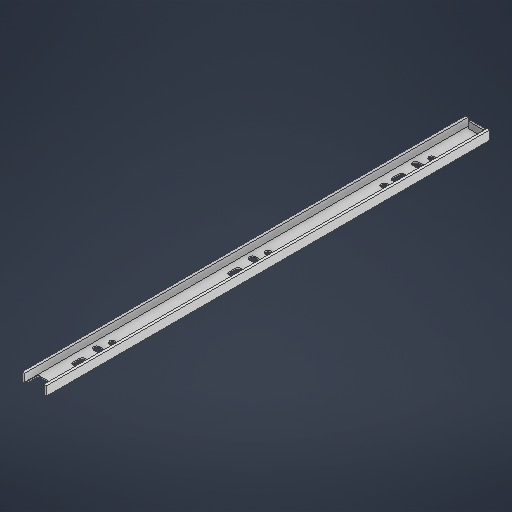
# Autodesk Inventor part: 3 часть направляшки 35
Saved by Autodesk Inventor 2025 (Build 290162000, 162)
## iProperties
Created: 2024-11-23
Part Number: 3 часть направляшки 35
Material: Типовые
Document SubType Name: Modeling
Designer: Phantom
Density: 1 g/cm^3
Appearance: По умолчанию
Author: Phantom
Autodesk Inventor part; units mm, degrees
ref_plane "YZ Plane" through (0, 0, 0) normal (1, 0, 0) x (0, 1, 0)
ref_plane "XZ Plane" through (0, 0, 0) normal (0, 1, 0) x (-1, 0, 0)
ref_plane "XY Plane" through (0, 0, 0) normal (0, 0, 1) x (1, 0, 0)
sketch "Эскиз1" plane through (0, 0, 0) normal (0, 0, 1) x (1, 0, 0)
  line L0 (0, 0) -> (24, 0)
  line L1 (24, 0) -> (24, 7)
  line L2 (24, 7) -> (0, 7)
  line L3 (0, 7) -> (0, 0)
  line L4 (0, 1) -> (24, 1)
  line L5 (2, 7) -> (2, 0)
  line L6 (22, 7) -> (22, 0)
  point P0 (0, 3.5)
  point P1 (12, 0)
  point P2 (2, 1)
  point P3 (22, 1)
  dimension "d0" = 24
  dimension "d1" = 7
  dimension "d2" = 2
  dimension "d3" = 2
  dimension "d4" = 1
  constraints: 14 end point, 4 perpendicular, 4 point on line, 2 midpoint, 2 parallel, 1 horizontal
  measures "d0" distance of L2.end L1.end
  measures "d1" distance of L1.end L0.end
  measures "d2" distance from line of point (0, 3.5) L5
  measures "d3" distance between parallel lines of L1 L6
  measures "d4" distance from line of point (12, 0) L4
extrude "Выдавливание1" add sketch "Эскиз1" along normal blind 397 contours L3 L4 L5 L0 | L5 L4 L6 L0 | L3 L2 L5 L4 | L6 L4 L1 L0 | L6 L2 L1 L4
sketch "Эскиз3" plane through (0, 0, 0) normal (0, -1, 0) x (1, 0, 0)
  line L0 (12.0033, 0) -> (12, 397)
  line L1 (22, 397) -> (2, 397) projected
  line L2 (24, 0) -> (24, 397) projected
  circle A0 centre (12.0005, 336) radius 2.25
  line L3 (12.0002, 366.75) -> (12.0003, 357.25) construction
  line L4 (9.7503, 364.5) -> (9.7503, 359.5)
  line L5 (14.2503, 359.5) -> (14.2503, 364.5)
  arc A1 (14.2503, 364.5) -> (9.7503, 364.5) centre (12.0003, 364.5) ccw
  arc A2 (9.7503, 359.5) -> (14.2503, 359.5) centre (12.0003, 359.5) ccw
  line L6 (16.7506, 346) -> (7.2506, 346) construction
  line L7 (14.5006, 348.25) -> (9.5006, 348.25)
  line L8 (9.5007, 343.75) -> (14.5007, 343.75)
  arc A3 (14.5007, 343.75) -> (14.5006, 348.25) centre (14.5006, 346) ccw
  arc A4 (9.5006, 348.25) -> (9.5007, 343.75) centre (9.5006, 346) ccw
  circle A5 centre (12.0013, 214) radius 2.25
  line L9 (12.001, 244.75) -> (12.0011, 235.25) construction
  line L10 (9.751, 242.5) -> (9.7511, 237.5)
  line L11 (14.2511, 237.5) -> (14.251, 242.5)
  arc A6 (14.251, 242.5) -> (9.751, 242.5) centre (12.001, 242.5) ccw
  arc A7 (9.7511, 237.5) -> (14.2511, 237.5) centre (12.0011, 237.5) ccw
  arc A8 (9.5014, 226.25) -> (9.5014, 221.75) centre (9.5014, 224) ccw
  line L12 (9.5014, 221.75) -> (14.5014, 221.75)
  line L13 (14.5014, 226.25) -> (9.5014, 226.25)
  line L14 (16.7514, 224) -> (7.2514, 224) construction
  arc A9 (14.5014, 221.75) -> (14.5014, 226.25) centre (14.5014, 224) ccw
  line L15 (9.5031, 93.75) -> (14.5031, 93.75)
  line L16 (16.7531, 96) -> (7.2531, 96) construction
  arc A10 (9.5031, 98.25) -> (9.5031, 93.75) centre (9.5031, 96) ccw
  line L17 (14.5031, 98.25) -> (9.5031, 98.25)
  arc A11 (14.5031, 93.75) -> (14.5031, 98.25) centre (14.5031, 96) ccw
  circle A12 centre (12.003, 86) radius 2.25
  arc A13 (9.7528, 109.5) -> (14.2528, 109.5) centre (12.0028, 109.5) ccw
  line L18 (14.2528, 109.5) -> (14.2528, 114.5)
  line L19 (9.7528, 114.5) -> (9.7528, 109.5)
  arc A14 (14.2528, 114.5) -> (9.7528, 114.5) centre (12.0028, 114.5) ccw
  line L20 (12.0027, 116.75) -> (12.0028, 107.25) construction
  circle A15 centre (12.0023, 123) radius 2.5
  point P0 (12.0003, 362)
  point P1 (12.0006, 346)
  point P2 (12.001, 240)
  point P3 (12.0014, 224)
  point P4 (12.0031, 96)
  point P5 (12.0028, 112)
  dimension "d47" = 4.5
  dimension "d49" = 9.5
  dimension "d50" = 4.5
  dimension "d51" = 9.5
  dimension "d52" = 4.5
  dimension "d53" = 10
  dimension "d54" = 16
  dimension "d55" = 70
  dimension "d56" = 4.5
  dimension "d57" = 9.5
  dimension "d58" = 4.5
  dimension "d59" = 9.5
  dimension "d60" = 4.5
  dimension "d61" = 10
  dimension "d62" = 16
  dimension "d63" = 138
  dimension "d64" = 4.5
  dimension "d65" = 9.5
  dimension "d66" = 4.5
  dimension "d67" = 9.5
  dimension "d68" = 4.5
  dimension "d69" = 10
  dimension "d70" = 16
  dimension "d71" = 138
  dimension "d72" = 5
  constraints: 50 end point, 36 point on circle, 24 tangent, 16 centre point, 16 point on line, 7 midpoint, 6 parallel
  measures "d47" diameter of A0
  measures "d49" distance of L3.start L3.end
  measures "d50" diameter of A2
  measures "d51" distance of L6.start L6.end
  measures "d52" diameter of A4
  measures "d53" distance of A0.centre point (12.001, 346)
  measures "d54" distance of point (12, 362) point (12.001, 346)
  measures "d55" diameter of point (12, 362) L1
  measures "d56" diameter of A5
  measures "d57" distance of L9.start L9.end
  measures "d58" diameter of A7
  measures "d59" distance of L14.start L14.end
  measures "d60" diameter of A8
  measures "d61" distance of A5.centre point (12.001, 224)
  measures "d62" distance of point (12.001, 240) point (12.001, 224)
  measures "d63" distance of point (12, 362) point (12.001, 224)
  measures "d64" diameter of A12
  measures "d65" distance of L20.start L20.end
  measures "d66" diameter of A13
  measures "d67" distance of L16.start L16.end
  measures "d68" diameter of A10
  measures "d69" distance of A12.centre point (12.003, 96)
  measures "d70" distance of point (12.003, 112) point (12.003, 96)
  measures "d71" distance of point (12.001, 224) A12.centre
  measures "d72" diameter of A15
extrude "Выдавливание2" cut sketch "Эскиз3" against normal blind 10
sketch "Эскиз4" plane through (0, 0, 0) normal (0, 0, -1) x (-1, 0, 0)
  line L0 (-2, 7) -> (0, 7) projected
  line L1 (-2, 1) -> (-2, 7) projected
  line L2 (-22, 1) -> (-2, 1) projected
  line L3 (-22, 7) -> (-22, 1) projected
  line L4 (-24, 7) -> (-22, 7) projected
  line L5 (-24, 0) -> (-24, 7) projected
  line L6 (0, 0) -> (-24, 0) projected
  line L7 (0, 7) -> (0, 0) projected
  line L8 (-12, 9) -> (-20, 9)
  line L9 (-20, 9) -> (-20, 0)
  line L10 (-12, 9) -> (-4, 9)
  line L11 (-4, 9) -> (-4, 0)
  point P0 (-20, 1)
  point P1 (-4, 1)
  constraints: 8 end point, 3 point on line, 2 perpendicular
extrude "Выдавливание3" add sketch "Эскиз4" against normal blind 1.5 contours L2 L9 L8 L10 L11
sketch "Эскиз5" plane through (0, 0, 0) normal (0, 0, -1) x (-1, 0, 0)
  line L0 (0, 0) -> (-24, 0) projected
  line L1 (-24, 7) -> (-21.5, 7)
  line L2 (-21.5, 7) -> (-21.5, 0)
  line L3 (-21.5, 0) -> (-24, 0)
  line L4 (-24, 0) -> (-24, 7)
  line L5 (0, 7) -> (-2.5, 7)
  line L6 (-2.5, 7) -> (-2.5, 0)
  line L7 (-2.5, 0) -> (0, 0)
  line L8 (0, 0) -> (0, 7)
  line L9 (-21.5, 7) -> (-19.5, 7)
  line L10 (-19.5, 7) -> (-19.5, 0)
  line L11 (-19.5, 0) -> (-21.5, 0)
  line L12 (-21.5, 0) -> (-21.5, 7)
  line L13 (-2.5, 7) -> (-4.5, 7)
  line L14 (-4.5, 7) -> (-4.5, 0)
  line L15 (-4.5, 0) -> (-2.5, 0)
  line L16 (-2.5, 0) -> (-2.5, 7)
  line L17 (-19.5, 0) -> (-17.5, 0)
  line L18 (-4.5, 0) -> (-6.5, 0)
  line L19 (-20, 9) -> (-4, 9) projected
  line L20 (-17.5, 0) -> (-6.5, 0)
  line L21 (-6.5, 0) -> (-6.5, 9)
  line L22 (-6.5, 9) -> (-17.5, 9)
  line L23 (-17.5, 9) -> (-17.5, 0)
  line L24 (-17.5, 7) -> (-21, 7)
  line L25 (-21, 7) -> (-21, 9)
  line L26 (-21, 9) -> (-17.5, 9)
  line L27 (-17.5, 9) -> (-17.5, 7)
  line L28 (-6.5, 7) -> (-4, 7)
  line L29 (-4, 7) -> (-4, 9)
  line L30 (-4, 9) -> (-6.5, 9)
  line L31 (-6.5, 9) -> (-6.5, 7)
  dimension "d36" = 2.5
  dimension "d37" = 2.5
  dimension "d38" = 2
  dimension "d39" = 2
  dimension "d40" = 2
  dimension "d41" = 2
  constraints: 60 end point, 14 parallel, 12 point on line, 7 horizontal, 7 perpendicular
  measures "d36" distance of L2.end L3.end
  measures "d37" distance of L7.end L6.end
  measures "d38" distance of L10.end L11.end
  measures "d39" distance of L15.end L14.end
  measures "d40" distance of L10.end L17.end
  measures "d41" distance of L14.end L18.end
extrude "Выдавливание4" cut sketch "Эскиз5" against normal through all contours L0 L6 L5 L8 | L0 L21 L28 L14 | L28 L21 L19 L29 L13 | L0 L10 L24 L23 | L24 L9 L25 L26 L19 L23 | L0 L4 L1 L2
sketch "Эскиз6" plane through (0, 0, 0) normal (0, 0, -1) x (-1, 0, 0)
  line L0 (-19.5, 0) -> (-21.5, 0) projected
  line L1 (-19.5, 0) -> (-19.5, 7) projected
  line L2 (-21.5, 0) -> (-19.5, 0)
  line L3 (-19.5, 0) -> (-19.5, 7)
  line L4 (-19.5, 7) -> (-21.5, 7)
  line L5 (-21.5, 7) -> (-21.5, 0)
  line L6 (-4.5, 1) -> (-4.5, 7) projected
  line L7 (-2.5, 0) -> (-4.5, 0) projected
  line L8 (-4.5, 7) -> (-2.5, 7)
  line L9 (-2.5, 7) -> (-2.5, 0)
  line L10 (-2.5, 0) -> (-4.5, 0)
  line L11 (-4.5, 0) -> (-4.5, 7)
  line L12 (-21.5, 1) -> (-2.5, 1)
  line L13 (-2.5, 1) -> (-2.5, 0)
  line L14 (-2.5, 0) -> (-21.5, 0)
  line L15 (-21.5, 0) -> (-21.5, 1)
  line L16 (-6.5, 0) -> (-6.5, 9) projected
  line L17 (-6.5, 1) -> (-6.5, 0)
  line L18 (-17.5, 1) -> (-6.5, 1) projected
  line L19 (-17.5, 9) -> (-17.5, 0) projected
  line L20 (-17.5, 1) -> (-17.5, 0)
  point P0 (0, 0)
  point P1 (-19.5, 1)
  constraints: 28 end point, 6 parallel, 3 horizontal, 3 perpendicular, 3 point on line, 2 collinear
extrude "Выдавливание5" add sketch "Эскиз6" against normal up to surface (397 mm away) contours L1 L12 L19 L14 | L12 L5 L4 L1 | L16 L12 L11 L14 | L6 L8 L9 L12
sketch "Эскиз7" plane through (2.5, 0, 0) normal (0, -1, 0) x (1, 0, 0)
  line L0 (0, 397) -> (19, 397) projected
  line L1 (9.5, 397) -> (2.5, 397)
  line L2 (9.5, 397) -> (16.5, 397)
  line L3 (16.5, 397) -> (16.5, 387)
  line L4 (16.5, 387) -> (2.5, 387)
  line L5 (2.5, 387) -> (2.5, 397)
  point P0 (-2.5, 0)
  dimension "d73" = 7
  dimension "d74" = 7
  dimension "d75" = 10
  constraints: 10 end point, 3 perpendicular, 2 point on line, 1 midpoint
  measures "d73" distance of L1.start L1.end
  measures "d74" distance of L1.start L2.end
  measures "d75" distance of L2.end L3.end
extrude "Выдавливание6" cut sketch "Эскиз7" against normal blind 10
fillet "Сопряжение1" radius 1 4 edges at (5, 0.5, 387) (19, 0.5, 387) (19, 0.5, 397) (5, 0.5, 397)
sketch "Эскиз8" plane through (0, 0, 0) normal (0, 0, -1) x (-1, 0, 0)
  line L0 (-6.5, 9) -> (-17.5, 9) projected
  line L1 (-17.5, 9) -> (-17.5, 1) projected
  line L2 (-6.5, 9) -> (-17.5, 9)
  line L3 (-17.5, 9) -> (-17.5, 6)
  line L4 (-17.5, 6) -> (-6.5, 6)
  line L5 (-6.5, 6) -> (-6.5, 9)
  point P0 (0, 0)
  constraints: 8 end point, 2 parallel, 1 horizontal, 1 perpendicular, 1 point on line
extrude "Выдавливание7" cut sketch "Эскиз8" against normal blind 10
sketch "Эскиз9" plane through (0, 0, 1.5) normal (0, 0, 1) x (1, 0, 0)
  line L0 (17.5, 6) -> (6.5, 6) projected
  line L1 (6.5, 6) -> (6.5, 1) projected
  line L2 (17.5, 1) -> (6.5, 1) projected
  line L3 (17.5, 1) -> (17.5, 6) projected
  point P0 (0, 0)
extrude "Выдавливание8" add sketch "Эскиз9" along normal blind 50
sketch "Эскиз10" plane through (0, 0, 0) normal (0, 0, -1) x (-1, 0, 0)
  line L0 (-30, 24) -> (32, 24)
  line L1 (32, 24) -> (32, -21)
  line L2 (32, -21) -> (-30, -21)
  line L3 (-30, -21) -> (-30, 24)
  point P0 (0, 0)
  constraints: 8 end point, 2 parallel, 1 horizontal, 1 perpendicular
extrude "Выдавливание9" cut sketch "Эскиз10" against normal blind 50
equation "\"d31\" = d61"
equation "\"d76\" = d61"
equation "\"d79\" = d61"
